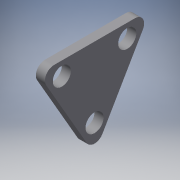
# Autodesk Inventor part: arm4_3
Saved by Autodesk Inventor 2016 (Build 200138000, 138)
## iProperties
Created: 2017-09-18
Part Number: arm4_3
Material: Generic
Document SubType Name: Modeling
Designer: student
Density: 1 g/cm^3
Appearance: Default
Author: student
Autodesk Inventor part; units mm, degrees
ref_plane "YZ Plane" through (0, 0, 0) normal (1, 0, 0) x (0, 1, 0)
ref_plane "XZ Plane" through (0, 0, 0) normal (0, 1, 0) x (-1, 0, 0)
ref_plane "XY Plane" through (0, 0, 0) normal (0, 0, 1) x (1, 0, 0)
sketch "Sketch1" plane through (0, 0, 0) normal (1, 0, 0) x (0, 1, 0)
  line L0 (13.7592, -3.5232) -> (-6.0382, 7.9068) construction
  line L1 (-6.0382, 7.9068) -> (13.7592, 19.3368) construction
  line L2 (13.7592, 19.3368) -> (13.7592, -3.5232) construction
  circle A0 centre (13.7592, 19.3368) radius 3.175
  circle A1 centre (13.7592, -3.5232) radius 3.175
  circle A2 centre (-6.0382, 7.9068) radius 3.175
  line L3 (-6.0382, 7.9068) -> (-15.5632, 7.9068) construction
  line L4 (-10.8007, 10.6565) -> (13.7592, 24.8361)
  line L5 (18.5217, 22.0865) -> (18.5217, -6.2728)
  line L6 (13.7592, -9.0224) -> (-10.8007, 5.1572)
  arc A3 (18.5217, 22.0865) -> (13.7592, 24.8361) centre (15.3467, 22.0865) ccw
  arc A4 (-10.8007, 10.6565) -> (-10.8007, 5.1572) centre (-9.2132, 7.9068) ccw
  arc A5 (13.7592, -9.0224) -> (18.5217, -6.2728) centre (15.3467, -6.2728) ccw
  point P0 (7.1601, 7.9068)
  point P1 (7.1601, 7.9068)
  point P2 (18.5217, 27.5857)
  point P3 (18.5217, -11.7721)
  dimension "d7" = 22.86
  dimension "d8" = 6.35
  dimension "d9" = 6.35
  dimension "d10" = 6.35
  dimension "d11" = 9.525
  dimension "d12" = 3.175
  constraints: 14 end point, 6 centre point, 6 point on circle, 6 point on line, 6 tangent, 4 coincident, 2 equal radius, 1 horizontal, 1 vertical, 14 other
  measures "d7" distance of L1.end L0.start
  measures "d8" diameter of A0
  measures "d9" diameter of A1
  measures "d10" diameter of A2
  measures "d11" distance of L3.start L3.end
  measures "d12" radius of A3
extrude "Extrusion1" add sketch "Sketch1" along normal blind 3.175
body "Solid1"
